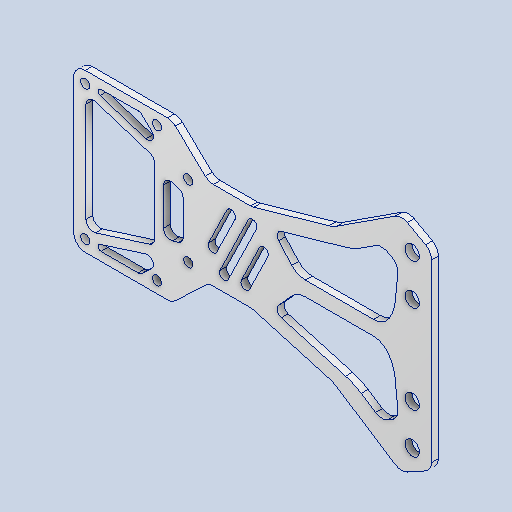
# Autodesk Inventor part: ShoulderBracket2
Saved by Autodesk Inventor 2023 (Build 270158000, 158)
## iProperties
Created: 2021-01-31
Part Number: ShoulderBracket2
Material: Aluminum 6061
Document SubType Name: Sheet Metal
Designer: valer
Density: 2.7 g/cm^3
Sheet Metal Rule: Default_mm
Appearance: Aluminum - Flat
Mass: 45.3627 g
Surface Area: 153.81 cm^2
Volume: 16.801 cm^3
Author: valer
Autodesk Inventor part; units mm, degrees
ref_plane "YZ Plane" through (0, 0, 0) normal (1, 0, 0) x (0, 1, 0)
ref_plane "XZ Plane" through (0, 0, 0) normal (0, 1, 0) x (-1, 0, 0)
ref_plane "XY Plane" through (0, 0, 0) normal (0, 0, 1) x (1, 0, 0)
sketch "Sketch1" plane through (0, 0, 0) normal (0, 0, 1) x (1, 0, 0)
  line L0 (-30.7756, 27.6953) -> (-17.6019, 15.2342)
  arc A0 (-30.7756, 27.6953) -> (-34.2665, 29.0848) centre (-34.2665, 24.0048) ccw
  line L1 (-70.3445, 29.0848) -> (-34.2665, 29.0848)
  arc A1 (-70.3445, 29.0848) -> (-75.4245, 24.0048) centre (-70.3445, 24.0048) ccw
  line L2 (-75.4245, -0.0806) -> (-75.4245, 24.0048)
  line L3 (-43.7214, 16.3936) -> (-63.813, 22.7947)
  arc A2 (-63.4274, 25.2748) -> (-63.813, 22.7947) centre (-63.4274, 24.0048) ccw
  line L4 (-63.4274, 25.2748) -> (-47.0956, 25.2748)
  arc A3 (-45.3502, 24.5801) -> (-47.0956, 25.2748) centre (-47.0956, 22.7348) ccw
  line L5 (-45.3502, 24.5801) -> (-41.2049, 20.659)
  arc A4 (-43.7214, 16.3936) -> (-41.2049, 20.659) centre (-42.9503, 18.8138) ccw
  arc A5 (-65.8672, 19.4505) -> (-70.006, 16.4253) centre (-66.831, 16.4253) ccw
  line L6 (-65.8672, 19.4505) -> (-41.9865, 11.8422)
  line L7 (-70.006, -0.0806) -> (-70.006, 16.4253)
  line L8 (-39.7753, 8.817) -> (-39.7753, -0.0806)
  arc A6 (-39.7753, 8.817) -> (-41.9865, 11.8422) centre (-42.9503, 8.817) ccw
  arc A7 (-17.6019, 15.2342) -> (-14.111, 13.8448) centre (-14.111, 18.9248) ccw
  line L9 (-14.111, 13.8448) -> (2.2031, 13.8448)
  line L10 (3.6033, 14.0416) -> (36.6802, 23.5262)
  arc A8 (2.2031, 13.8448) -> (3.6033, 14.0416) centre (2.2031, 18.9248) ccw
  line L11 (40.0965, 25.0831) -> (65.7679, 41.7543)
  arc A9 (36.6802, 23.5262) -> (40.0965, 25.0831) centre (33.1796, 35.7342) ccw
  arc A10 (70.9975, 41.9369) -> (65.7679, 41.7543) centre (68.5347, 37.4939) ccw
  line L12 (70.9975, 41.9369) -> (79.0399, 37.479)
  arc A11 (81.6571, 33.0359) -> (79.0399, 37.479) centre (76.5771, 33.0359) ccw
  line L13 (81.6571, 33.0359) -> (81.6571, -0.0806)
  line L14 (15.7144, 10.9085) -> (43.9523, 19.0056)
  line L15 (50.785, 22.1194) -> (57.1081, 26.2257)
  arc A12 (43.9523, 19.0056) -> (50.785, 22.1194) centre (36.9512, 43.4216) ccw
  arc A13 (15.7144, 10.9085) -> (14.527, 6.7673) centre (16.4146, 8.4669) ccw
  line L16 (22.7094, -2.3202) -> (14.527, 6.7673)
  line L17 (66.8628, 20.3613) -> (65.2538, 5.1137)
  arc A14 (66.8628, 20.3613) -> (64.2734, 25.3353) centre (61.8106, 20.8923) ccw
  line L18 (62.3377, 26.4083) -> (64.2734, 25.3353)
  arc A15 (62.3377, 26.4083) -> (57.1081, 26.2257) centre (59.8749, 21.9652) ccw
  circle A16 centre (73.1904, 31.6694) radius 3.175
  circle A17 centre (73.1904, 13.8894) radius 3.175
  circle A18 centre (-38.8445, 24.0048) radius 2
  circle A19 centre (-25.0945, 10.2548) radius 2
  circle A20 centre (-25.0945, -21.2452) radius 2
  circle A21 centre (-70.3445, 24.0048) radius 2
  line L19 (-75.4245, -0.0806) -> (81.6571, -0.0806) construction
  line L20 (-42.9503, 18.8138) -> (-42.9503, 8.817) construction
  line L21 (-25.0945, 10.2548) -> (-25.0945, -21.2452) construction
  line L22 (-90, -5.4952) -> (-25.0945, -5.4952) construction
  circle A22 centre (-70.3445, -34.9952) radius 2
  arc A23 (-75.4245, -34.9952) -> (-70.3445, -40.0752) centre (-70.3445, -34.9952) ccw
  line L23 (-75.4245, -10.9098) -> (-75.4245, -34.9952)
  line L24 (-70.3445, -40.0752) -> (-34.2665, -40.0752)
  circle A24 centre (-38.8445, -34.9952) radius 2
  arc A25 (-34.2665, -40.0752) -> (-30.7756, -38.6858) centre (-34.2665, -34.9952) ccw
  line L25 (-30.7756, -38.6858) -> (-17.6019, -26.2247)
  arc A26 (-14.111, -24.8352) -> (-17.6019, -26.2247) centre (-14.111, -29.9152) ccw
  line L26 (-14.111, -24.8352) -> (2.2031, -24.8352)
  line L27 (-75.4245, -0.0806) -> (-75.4245, -10.9098)
  arc A27 (-63.813, -33.7851) -> (-63.4274, -36.2652) centre (-63.4274, -34.9952) ccw
  arc A28 (-70.006, -27.4157) -> (-65.8672, -30.4409) centre (-66.831, -27.4157) ccw
  line L28 (-70.006, -0.0806) -> (-70.006, -27.4157)
  line L29 (-63.4274, -36.2652) -> (-47.0956, -36.2652)
  line L30 (-65.8672, -30.4409) -> (-41.9865, -22.8326)
  line L31 (-43.7214, -27.384) -> (-63.813, -33.7851)
  arc A29 (-47.0956, -36.2652) -> (-45.3502, -35.5705) centre (-47.0956, -33.7252) ccw
  line L32 (-45.3502, -35.5705) -> (-41.2049, -31.6495)
  arc A30 (-41.9865, -22.8326) -> (-39.7753, -19.8075) centre (-42.9503, -19.8075) ccw
  arc A31 (-41.2049, -31.6495) -> (-43.7214, -27.384) centre (-42.9503, -29.8042) ccw
  line L33 (-39.7753, -19.8075) -> (-39.7753, -0.0806)
  arc A32 (3.6033, -25.032) -> (2.2031, -24.8352) centre (2.2031, -29.9152) ccw
  line L34 (3.6033, -25.032) -> (36.6802, -34.5166)
  arc A33 (79.0399, -48.4694) -> (81.6571, -44.0263) centre (76.5771, -44.0263) ccw
  line L35 (70.9975, -52.9274) -> (79.0399, -48.4694)
  circle A34 centre (73.1904, -42.6598) radius 3.175
  line L36 (40.0965, -36.0736) -> (65.7679, -52.7447)
  arc A35 (65.7679, -52.7447) -> (70.9975, -52.9274) centre (68.5347, -48.4843) ccw
  circle A36 centre (73.1904, -24.8798) radius 3.175
  arc A37 (40.0965, -36.0736) -> (36.6802, -34.5166) centre (33.1796, -46.7247) ccw
  line L37 (81.6571, -44.0263) -> (81.6571, -10.9098)
  line L38 (81.6571, -10.9098) -> (81.6571, -0.0806)
  line L39 (65.2538, 5.1137) -> (60.6034, -2.3202)
  line L40 (60.6034, -2.3202) -> (22.7094, -2.3202)
  line L41 (62.3377, -37.3987) -> (64.2734, -36.3258)
  arc A38 (64.2734, -36.3258) -> (66.8628, -31.3517) centre (61.8106, -31.8827) ccw
  arc A39 (57.1081, -37.2161) -> (62.3377, -37.3987) centre (59.8749, -32.9557) ccw
  line L42 (66.8628, -31.3517) -> (65.2538, -16.1042)
  line L43 (50.785, -33.1098) -> (57.1081, -37.2161)
  arc A40 (50.785, -33.1098) -> (43.9523, -29.996) centre (36.9512, -54.412) ccw
  arc A41 (14.527, -17.7577) -> (15.7144, -21.8989) centre (16.4146, -19.4573) ccw
  line L44 (22.7094, -8.6702) -> (14.527, -17.7577)
  line L45 (15.7144, -21.8989) -> (43.9523, -29.996)
  line L46 (65.2538, -16.1042) -> (60.6034, -8.6702)
  line L47 (60.6034, -8.6702) -> (22.7094, -8.6702)
  point P0 (0, 0)
  dimension "d0" = 3.175
  dimension "d1" = 3.175
  dimension "d2" = 2.54
  dimension "d3" = 1.27
  dimension "d4" = 2.54
  dimension "d5" = 4
  dimension "d6" = 72.328
  dimension "d11" = 3.81
  dimension "d12" = 16.3318
  dimension "d13" = 3.4035
  dimension "d14" = 7.5795
  dimension "d16" = 3.81
  dimension "d18" = 5.4186
  dimension "d29" = 6.35
  dimension "d30" = 6.35
  dimension "d31" = 16.4032
  dimension "d32" = 21.0537
  measures "d0" radius of A5
  measures "d1" radius of A6
  measures "d2" radius of A4
  measures "d3" radius of A2
  measures "d4" radius of A3
  measures "d5" diameter of A21
  measures "d6" angle of L7 L6
  measures "d11" distance between parallel lines of L1 L4
  measures "d12" distance of L4.start L4.end
  measures "d13" horizontal distance of A5.centre A2.centre
  measures "d14" vertical distance of A2.centre A5.centre
  measures "d16" distance between parallel lines of L6 L3
  measures "d18" distance between parallel lines of L2 L7
  measures "d29" distance between parallel lines of L10 L14
  measures "d30" distance between parallel lines of L47 L40
  measures "d31" distance from line of L13 L17.end
  measures "d32" distance from line of L38 L39.end
extrude "Plate1" add sketch "Sketch1" along normal blind 3
sketch "Sketch2" plane through (0, 0, 3) normal (0, 0, 1) x (1, 0, 0)
  line L0 (-35.9653, 6.8061) -> (-27.288, 4.1313)
  line L1 (-27.288, 4.1313) -> (-27.288, -15.1217)
  line L2 (-27.288, -15.1217) -> (-35.9653, -17.7966)
  line L3 (-35.9653, -17.7966) -> (-35.9653, 6.8061)
  line L4 (-39.7753, 8.817) -> (-39.7753, -19.8075) construction
  line L5 (-39.7753, -19.8075) -> (-39.7753, 8.817) construction
  line L6 (-39.7753, -5.4952) -> (-35.9653, -5.4952) construction
  line L7 (-65.8672, 19.4505) -> (-41.9865, 11.8422) projected
  line L8 (-43.7214, 16.3936) -> (-63.813, 22.7947) projected
  point P0 (0, 0)
  dimension "d20" = 3.81
  dimension "d21" = 3.81
  dimension "d22" = 72.868
  dimension "d23" = 72.868
  constraints: 10 end point, 2 midpoint, 1 equal length, 1 parallel, 1 perpendicular, 1 vertical
  measures "d20" distance between parallel lines of L7 L8
  measures "d21" distance between parallel lines of L4 L3
  measures "d22" angle of L0 L3
  measures "d23" angle of L3 L2
extrude "Extrusion1" cut sketch "Sketch2" against normal blind 10
fillet "Fillet1" radius 3 4 edges at (-35.9653, 6.8061, 1.5) (-27.288, 4.1313, 1.5) (-27.288, -15.1217, 1.5) (-35.9653, -17.7966, 1.5)
fillet "Fillet2" radius 16 2 edges at (65.2538, 5.1137, 1.5) (65.2538, -16.1042, 1.5)
fillet "Fillet3" radius 8 4 edges at (60.6034, -2.3202, 1.5) (22.7094, -2.3202, 1.5) (22.7094, -8.6702, 1.5) (60.6034, -8.6702, 1.5)
sketch "Sketch4" plane through (0, 0, 3) normal (0, 0, 1) x (1, 0, 0)
  line L0 (-14.3978, -10.2253) -> (-6.3628, 6.2488) construction
  line L1 (-12.6002, -11.102) -> (-4.5653, 5.3721)
  line L2 (-8.1604, 7.1255) -> (-16.1954, -9.3486)
  arc A0 (-16.1954, -9.3486) -> (-12.6002, -11.102) centre (-14.3978, -10.2253) ccw
  arc A1 (-4.5653, 5.3721) -> (-8.1604, 7.1255) centre (-6.3628, 6.2488) ccw
  line L3 (-9.3916, -18.2104) -> (3.0116, 7.2199) construction
  line L4 (-11.1892, -17.3336) -> (1.214, 8.0967)
  line L5 (4.8092, 6.3432) -> (-7.594, -19.0871)
  arc A2 (-11.1892, -17.3336) -> (-7.594, -19.0871) centre (-9.3916, -18.2104) ccw
  arc A3 (4.8092, 6.3432) -> (1.214, 8.0967) centre (3.0116, 7.2199) ccw
  line L6 (-0.0171, -17.2392) -> (8.0179, -0.7651) construction
  line L7 (-1.8147, -16.3625) -> (6.2203, 0.1116)
  line L8 (9.8155, -1.6419) -> (1.7805, -18.116)
  arc A4 (-1.8147, -16.3625) -> (1.7805, -18.116) centre (-0.0171, -17.2392) ccw
  arc A5 (9.8155, -1.6419) -> (6.2203, 0.1116) centre (8.0179, -0.7651) ccw
  circle A6 centre (-25.0945, 10.2548) radius 2 projected
  line L9 (-27.288, 1.9168) -> (-27.288, -12.9072) projected
  line L10 (-10.3803, -1.9882) -> (4.0004, -9.0022) construction
  line L11 (-14.111, 13.8448) -> (2.2031, 13.8448) projected
  line L12 (2.2031, -24.8352) -> (-14.111, -24.8352) projected
  point P0 (0, 0)
  point P1 (-3.19, -5.4952)
  point P2 (-3.19, -5.4952)
  dimension "d37" = 26
  dimension "d38" = 6.6248
  dimension "d39" = 6.6248
  dimension "d40" = 4
  dimension "d41" = 4
  constraints: 26 end point, 12 point on circle, 12 tangent, 6 centre point, 6 midpoint, 6 parallel, 3 equal radius, 1 perpendicular
  measures "d37" angle of L9 L0
  measures "d38" distance from line of L11 L3.end
  measures "d39" distance from line of L12 L3.start
  measures "d40" distance between parallel lines of L4 L1
  measures "d41" distance between parallel lines of L7 L5
extrude "Extrusion3" cut sketch "Sketch4" against normal blind 10 contours A0 L2 A1 L1 | L4 A3 L5 A2 | L7 A5 L8 A4
equation "\"d21\" = d20"
equation "\"d23\" = d22"
equation "\"d19\" = Thickness"
equation "\"BendRadius\" = Thickness"
equation "\"BendReliefWidth\" = Thickness"
equation "\"BendReliefDepth\" = 0.5 * Thickness"
equation "\"CornerReliefSize\" = 4 * Thickness"
equation "\"MinimumRemnant\" = 2 * Thickness"
equation "\"TransitionRadius\" = BendRadius"
equation "\"JacobiRadiusSize\" = BendRadius"
equation "\"GapSize\" = Thickness"
equation "\"Thickness\" = 3"
body "Solid1"
